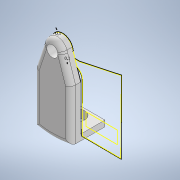
# Autodesk Inventor part: Tool Head Clamp
Saved by Autodesk Inventor 2022.2 (Build 262287000, 287)
## iProperties
Created: 2022-08-16
Part Number: Tool Head Clamp
Material: Generic
Document SubType Name: Modeling
Designer: Ilewicz
Density: 1 g/cm^3
Appearance: Default
Author: Ilewicz
Autodesk Inventor part; units mm, degrees
ref_plane "YZ Plane" through (0, 0, 0) normal (1, 0, 0) x (0, 1, 0)
sketch "Sketch1" plane through (0, 0, 0) normal (0, 0, 1) x (1, 0, 0)
  circle A0 centre (0, 8.95) radius 1.09 projected
  arc A1 (1.662, 7.8375) -> (-0.0143, 6.9501) centre (0, 8.95) ccw projected
  arc A2 (1.8983, 9.5797) -> (-1.8983, 9.5797) centre (0, 8.95) ccw
  line L0 (3.6, 4.45) -> (3.6, -5.6116)
  arc A3 (-3.6, -5.6116) -> (3.6, -5.6116) centre (0, 8.95) ccw
  circle A4 centre (0, 8.95) radius 4.08 projected
  circle A5 centre (0, 8.95) radius 15 projected
  line L1 (2.5, -0.05) -> (2.5, 4.45) projected
  line L2 (2.5, 4.45) -> (3.6, 4.45) projected
  line L3 (3.6, 4.45) -> (3.6, -4.45) projected
  line L4 (3.6, -4.45) -> (-3.6, -4.45) projected
  line L5 (-3.6, -4.45) -> (-3.6, 4.45) projected
  line L6 (-3.6, 4.45) -> (-2.5, 4.45) projected
  line L7 (-2.5, 4.45) -> (-2.5, -0.05) projected
  line L8 (-3.6, -5.6116) -> (-3.6, 4.45)
  line L9 (-3.6, 4.45) -> (-1.8983, 9.5797)
  line L10 (3.6, 4.45) -> (1.8983, 9.5797)
  line L11 (-2.5, -0.05) -> (2.5, -0.05) projected
  point P0 (0, 0)
  point P1 (-1.8983, 9.5797)
  constraints: 8 end point, 6 point on circle, 3 tangent, 2 centre point, 2 collinear, 1 concentric
extrude "Extrusion1" add sketch "Sketch1" along normal blind 2 contours L10 A4 L9 A1 | L10 L2 L1 L11 L7 L6 L9 A4 | L0 L4 L5 L6 L7 L11 L1 L2 | L0 A3 L8 L4 picked at (1.9915, 8.1578)
sketch "Sketch2" plane through (0, 0, 0) normal (0, 0, -1) x (-1, 0, 0)
  line L0 (-3.6, -4.45) -> (3.6, -4.45) projected
  line L1 (-3.6, 4.45) -> (-1.8983, 9.5797) projected
  line L2 (-3.6, -5.6116) -> (-3.6, 4.45) projected
  arc A0 (-3.6, -5.6116) -> (3.6, -5.6116) centre (0, 8.95) ccw projected
  line L3 (3.6, 4.45) -> (3.6, -5.6116) projected
  line L4 (1.8983, 9.5797) -> (3.6, 4.45) projected
  arc A1 (1.8983, 9.5797) -> (-1.8983, 9.5797) centre (0, 8.95) ccw projected
  circle A2 centre (0, 8.95) radius 1.09 projected
  point P0 (0, 0)
ref_plane "Work Plane1" through (-15.2152, -6.2652, -4.8) normal (0, 0, 1) x (1, 0, 0)
extrude "Extrusion2" add sketch "Sketch2" along normal up to surface (4.8 mm away) contours L0 L3 A0 L2
sketch "Sketch3" plane through (-3.6, -4.45, 0) normal (0, 1, 0) x (1, 0, 0)
  circle A0 centre (3.6, 2.8) radius 1.6 projected
  point P0 (3.6, 0)
extrude "Extrusion3" cut sketch "Sketch3" against normal blind 10
fillet "Fillet1" radius 1 6 edges at (2.7491, 7.0149, 2) (3.6, -0.5808, 2) (0, -6.05, 2) (-3.6, -0.5808, 2) (-2.7491, 7.0149, 2) (0, 10.95, 2)
sketch "Sketch4" plane through (0, 0, 0) normal (0, 0, -1) x (-1, 0, 0)
  point P0 (0, 0)
sketch "Sketch5" plane through (0, 0, 0) normal (0, 0, -1) x (-1, 0, 0)
  line L0 (-3.6, 4.45) -> (3.6, 4.45) projected
  arc A0 (0.0143, 6.9501) -> (-1.662, 7.8375) centre (0, 8.95) ccw projected
  circle A1 centre (0, 8.95) radius 1.09 projected
  line L1 (-3.8923, -4.5783) -> (-11.4921, -4.6328) projected
  line L2 (-11.4921, -4.6328) -> (-11.5941, 9.5788) projected
  line L3 (-3.3887, 7.8251) -> (-11.5941, 9.5788) projected
  line L4 (-1.662, 7.8375) -> (-3.3887, 7.8251) projected
  arc A2 (0.0143, 6.9501) -> (-1.662, 7.8375) centre (0, 8.95) ccw projected
  line L5 (0.0143, 6.9501) -> (-1.9749, 6.9358) projected
  arc A3 (-1.9749, 6.9358) -> (-3.9605, 4.9215) centre (-1.9605, 4.9358) ccw projected
  line L6 (-3.9605, 4.9215) -> (-3.8923, -4.5783) projected
  line L7 (-10.8065, -2.6278) -> (-4.6067, -2.5833) projected
  line L8 (-4.6067, -2.5833) -> (-4.6246, -0.0834) projected
  line L9 (-4.6246, -0.0834) -> (-10.8244, -0.1279) projected
  line L10 (-10.8244, -0.1279) -> (-10.8065, -2.6278) projected
  line L11 (-3.6, 4.45) -> (-1.8983, 9.5797) projected
  line L12 (-3.6, 4.45) -> (-2.8435, 6.7304)
  line L13 (1.8983, 9.5797) -> (2.0348, 9.1681) projected
  line L14 (3.6, 4.45) -> (1.8983, 9.5797)
  arc A4 (0.0151, 6.8501) -> (-1.7451, 7.7818) centre (0, 8.95) ccw
  line L15 (0.0151, 6.8501) -> (-1.9742, 6.8358)
  arc A5 (-1.9742, 6.8358) -> (-3.8605, 4.9222) centre (-1.9605, 4.9358) ccw
  line L16 (-3.8605, 4.9222) -> (-3.7916, -4.6775)
  line L17 (-3.7916, -4.6775) -> (-11.5914, -4.7335)
  line L18 (-11.5914, -4.7335) -> (-11.695, 9.7026)
  line L19 (-11.695, 9.7026) -> (-3.3785, 7.9252)
  line L20 (-3.3785, 7.9252) -> (-1.6627, 7.9375)
  point P0 (0, 0)
  point P1 (2.0999, 8.972)
  point P2 (0.0151, 6.8501)
  point P3 (-2.8889, 6.5936)
  dimension "d7" = 0.1
  dimension "d8" = 0.1
  constraints: 16 end point, 5 point on circle, 2 centre point, 1 collinear, 1 point on line, 1 tangent, 6 other
  measures "d7" radial gap between concentric circles of A0 A4
  measures "d8" distance between parallel lines of L5 L15
ref_plane "Work Plane2" through (-2.5323, -0.0859, -0.8) normal (0, 0, -1) x (0, 1, 0)
extrude "Extrusion4" add sketch "Sketch5" along normal up to surface (0.8 mm away) contours L11 A5 L15 A4 L14 L0
body "Solid1"
